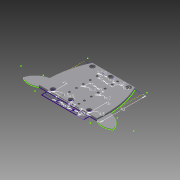
# Autodesk Inventor part: Piece
Saved by Autodesk Inventor 2014 SP1 (Build 180222100, 222)
## iProperties
Created: 2015-03-21
Part Number: Piece
Material: Generic
Document SubType Name: Modeling
Designer: Erin
Density: 1 g/cm^3
Appearance: Default
Author: Erin
Autodesk Inventor part; units mm, degrees
ref_plane "YZ Plane" through (0, 0, 0) normal (1, 0, 0) x (0, 1, 0)
ref_plane "XZ Plane" through (0, 0, 0) normal (0, 1, 0) x (-1, 0, 0)
ref_plane "XY Plane" through (0, 0, 0) normal (0, 0, 1) x (1, 0, 0)
sketch "Block1" plane through (0, 0, 0) normal (0, 0, 1) x (1, 0, 0)
  line L0 (22.5674, 54.9733) -> (22.5674, 26.9733) construction
  line L1 (62.5674, 54.9733) -> (62.5674, 26.9733) construction
  line L2 (42.5674, 54.9733) -> (42.5674, 26.9733) construction
  arc A0 (22.5674, 54.9733) -> (16.0189, 31.9733) centre (39.6923, 37.6653) ccw
  arc A1 (69.116, 31.9733) -> (62.5674, 54.9733) centre (45.4425, 37.6653) ccw
  line L3 (67.5674, 31.9733) -> (69.116, 31.9733)
  line L4 (22.5674, 54.9733) -> (62.5674, 54.9733)
  arc A2 (3.175, 28.049) -> (16.0189, 31.9733) centre (7.7246, 36.1392) ccw
  arc A3 (15.3685, 38.7512) -> (3.175, 28.049) centre (13.5542, 28.5209) ccw
  arc A4 (69.116, 31.9733) -> (81.9598, 28.049) centre (77.4102, 36.1392) ccw
  arc A5 (81.9598, 28.049) -> (69.7664, 38.7512) centre (71.5807, 28.5209) ccw
  line L5 (17.5674, 54.9733) -> (67.5674, 54.9733) construction
  line L6 (67.5674, 54.9733) -> (67.5674, 31.9733) construction
  line L7 (67.5674, 31.9733) -> (16.0189, 31.9733)
  line L8 (17.5674, 31.9733) -> (17.5674, 54.9733) construction
  line L9 (22.5674, 31.9733) -> (62.5674, 31.9733)
  line L10 (62.5674, 31.9733) -> (62.5674, 26.9733)
  line L11 (62.5674, 26.9733) -> (22.5674, 26.9733)
  line L12 (22.5674, 26.9733) -> (22.5674, 31.9733)
  circle A6 centre (35.5674, 51.6287) radius 1
  circle A7 centre (49.5674, 51.6287) radius 1
  line L13 (22.5674, 29.4733) -> (62.5674, 29.4733) construction
  circle A8 centre (35.5674, 29.4733) radius 1
  circle A9 centre (49.5674, 29.4733) radius 1
  point P0 (42.5377, 37.3132)
  point P1 (42.5674, 31.9733)
  point P2 (42.5674, 31.9733)
  point P3 (17.5674, 26.9733)
  point P4 (67.5674, 26.9733)
  dimension "d0" = 23
  dimension "d1" = 5
  dimension "d2" = 40
  dimension "d3" = 2
  dimension "d4" = 2
  dimension "d5" = 7
  dimension "d6" = 7
  dimension "d7" = 2
  dimension "d8" = 2
  dimension "d9" = 7
  dimension "d10" = 7
  measures "d0" distance of L5.end L3.start
  measures "d1" distance of L9.end L1.end
  measures "d2" distance of L9.start L9.end
  measures "d3" diameter of A6
  measures "d4" diameter of A7
  measures "d5" distance from line of A6.centre L2
  measures "d6" distance from line of A7.centre L2
  measures "d7" diameter of A8
  measures "d8" diameter of A9
  measures "d9" distance from line of A8.centre L2
  measures "d10" distance from line of A9.centre L2
sketch "Sketch1" plane through (0, 0, 0) normal (0, 0, 1) x (1, 0, 0)
  line L0 (-20, 21.5) -> (-20, -26.5) construction
  line L1 (20, 21.5) -> (20, -26.5) construction
  line L2 (0, 21.5) -> (0, -26.5) construction
  line L3 (27.1698, -21.5) -> (25.1885, -21.5)
  line L4 (-20, 21.5) -> (20, 21.5)
  line L5 (-27.1698, 21.5) -> (27.1698, 21.5) construction
  line L6 (27.1698, 21.5) -> (27.1698, -21.5) construction
  line L7 (27.1698, -21.5) -> (-27.1698, -21.5)
  line L8 (-27.1698, -21.5) -> (-27.1698, 21.5) construction
  line L9 (-20, -21.5) -> (20, -21.5)
  line L10 (20, -21.5) -> (20, -26.5)
  line L11 (20, -26.5) -> (-20, -26.5)
  line L12 (-20, -26.5) -> (-20, -21.5)
  circle A0 centre (-7, 18.1554) radius 1
  circle A1 centre (7, 18.1554) radius 1
  line L13 (-20, -24) -> (20, -24) construction
  circle A2 centre (-7, -24) radius 1
  circle A3 centre (7, -24) radius 1
  circle A4 centre (-17, -18.5) radius 2.25
  circle A5 centre (17, -18.5) radius 2.25
  circle A6 centre (0, -18.5) radius 2.25
  line L14 (-27.1698, 0) -> (27.1698, 0) construction
  circle A7 centre (-7, 0) radius 1
  circle A8 centre (7, 0) radius 1
  circle A9 centre (-7, -18.1554) radius 1
  circle A10 centre (7, -18.1554) radius 1
  arc A11 (-20, 21.5) -> (-27.1698, -21.5) centre (52.9621, -12.7633) ccw
  arc A12 (27.1698, -21.5) -> (20, 21.5) centre (-52.9621, -12.7633) ccw
  arc A13 (-42.2904, -21.5) -> (-27.1698, -21.5) centre (-34.7301, -9.753) ccw
  arc A14 (-27.5757, -9.4306) -> (-42.2904, -21.5) centre (-25.9265, -26.4458) ccw
  arc A15 (27.1698, -21.5) -> (42.2904, -21.5) centre (34.7301, -9.753) ccw
  arc A16 (42.2904, -21.5) -> (27.5757, -9.4306) centre (25.9265, -26.4458) ccw
  point P0 (0, 0)
  point P1 (0, -21.5)
  point P2 (0, -21.5)
  point P3 (-27.9814, 24.963)
  point P4 (27.9814, 24.963)
  point P5 (0, -2.5)
  point P6 (0, 0)
  dimension "d12" = 43
  dimension "d13" = 5
  dimension "d14" = 40
  dimension "d15" = 2
  dimension "d16" = 2
  dimension "d17" = 7
  dimension "d18" = 7
  dimension "d19" = 2
  dimension "d20" = 2
  dimension "d21" = 7
  dimension "d22" = 7
  dimension "d24" = 4.5
  dimension "d25" = 4.5
  dimension "d26" = 3
  dimension "d27" = 3
  dimension "d28" = 3
  dimension "d29" = 3
  dimension "d34" = 4.5
  dimension "d35" = 3
  dimension "d38" = 3.3446
  dimension "d39" = 3.3446
  dimension "d40" = 2
  dimension "d41" = 2
  dimension "d42" = 7
  dimension "d43" = 7
  constraints: 30 end point, 17 centre point, 13 point on circle, 10 midpoint, 7 point on line, 7 symmetric about line, 6 parallel, 3 horizontal, 3 perpendicular, 2 collinear, 1 coincident, 1 vertical, 5 other
  measures "d12" distance of L5.end L3.start
  measures "d13" distance of L9.end L1.end
  measures "d14" distance of L9.start L9.end
  measures "d15" diameter of A0
  measures "d16" diameter of A1
  measures "d17" distance from line of A0.centre L2
  measures "d18" distance from line of A1.centre L2
  measures "d19" diameter of A2
  measures "d20" diameter of A3
  measures "d21" distance from line of A2.centre L2
  measures "d22" distance from line of A3.centre L2
  measures "d24" diameter of A4
  measures "d25" diameter of A5
  measures "d26" distance from line of A4.centre L0
  measures "d27" distance from line of A5.centre L1
  measures "d28" distance from line of A4.centre L9
  measures "d29" distance from line of A5.centre L7
  measures "d34" diameter of A6
  measures "d35" distance from line of A6.centre L9
  measures "d38" distance from line of A0.centre L4
  measures "d39" distance from line of A1.centre L4
  measures "d40" diameter of A7
  measures "d41" diameter of A8
  measures "d42" distance from line of A7.centre L2
  measures "d43" distance from line of A8.centre L2
extrude "Extrusion1" add sketch "Sketch1" along normal blind 2 contours L3 L7 A11 L4 A12 | A4 | A5 | A6 | A7 | A8
extrude "Extrusion2" add sketch "Sketch1" along normal blind 0.6 contours A13 A14 A11
mirror "Mirror1" about plane through (0, 0, 0) normal (1, 0, 0) of "Extrusion2"
extrude "Extrusion3" cut sketch "Sketch1" along normal blind 5 contours A4 | A5 | A6
mirror "Mirror2" about plane through (0, 0, 0) normal (0, 1, 0) of "Extrusion3"
extrude "Extrusion4" cut sketch "Sketch1" along normal blind 10 contours A7 | A8
pattern_linear "Rectangular Pattern1" count 3 spacing 6.5 along (0, 1, 0) count 3 spacing 6.5 along (0, -1, 0) of "Extrusion4"
equation "\"d3\" = d11"
equation "\"d4\" = d11"
equation "\"d7\" = d11"
equation "\"d8\" = d11"
equation "\"d15\" = fishing"
equation "\"d16\" = fishing"
equation "\"d19\" = fishing"
equation "\"d20\" = fishing"
equation "\"d40\" = fishing"
equation "\"d41\" = fishing"
equation "\"d11\" = 2"
equation "\"d23\" = 2"
equation "\"fishing\" = 2"
body "Solid1"
